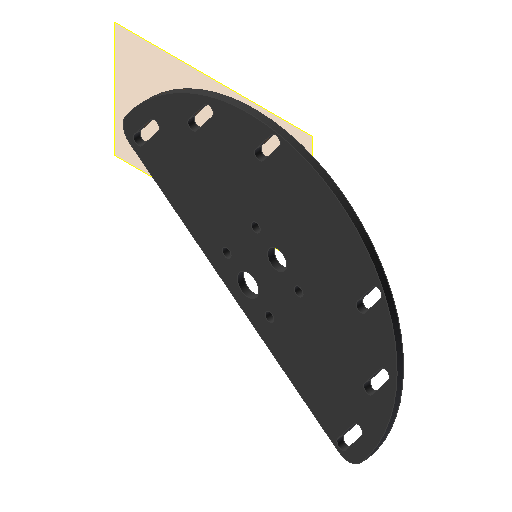
# Autodesk Inventor part: Anglerfish_Lightplate_Tosslink_adjuster_flipped
Saved by Autodesk Inventor 2022 (Build 260153000, 153)
## iProperties
Created: 2022-10-26
Part Number: Anglerfish_Lightplate_Tosslink_adjuster_flipped
Material: Generisch
Document SubType Name: Modeling
Designer: diederichbenedict
Density: 1 g/cm^3
Appearance: Vorgabe
Author: diederichbenedict
Autodesk Inventor part; units mm, degrees
ref_plane "YZ Plane" through (0, 0, 0) normal (1, 0, 0) x (0, 1, 0)
ref_plane "XZ Plane" through (0, 0, 0) normal (0, 1, 0) x (-1, 0, 0)
ref_plane "XY Plane" through (0, 0, 0) normal (0, 0, 1) x (1, 0, 0)
ref_plane "Arbeitsebene1" through (0, 0, 0) normal (0, 0, 1) x (1, 0, 0)
sketch "Skizze1" plane through (0, 0, 0) normal (0, 0, 1) x (1, 0, 0)
  line L0 (39.3233, 58.7442) -> (31.1975, 48.5587) projected
  arc A0 (20.3661, 6.7006) -> (31.1975, 48.5587) centre (0, 34.301) ccw projected
  line L1 (20.3661, 6.7006) -> (24.3422, 1.3125) projected
  arc A1 (24.3422, 1.3125) -> (31.7994, 0.6471) centre (28.3654, 4.2814) ccw projected
  arc A2 (31.7994, 0.6471) -> (39.3233, 58.7442) centre (0, 34.301) ccw projected
  circle A3 centre (37.5836, 49.0481) radius 1.4 projected
  circle A4 centre (39.9219, 28.2806) radius 1.4 projected
  circle A5 centre (31.5631, 9.1262) radius 1.4 projected
  line L2 (6.9617, 67.8882) -> (15.0883, 78.0746) projected
  arc A6 (15.0883, 78.0746) -> (-39.8826, 57.8205) centre (0, 34.301) ccw projected
  arc A7 (-39.8826, 57.8205) -> (-37.5755, 50.698) centre (-35.5757, 55.2807) ccw projected
  line L3 (-37.5755, 50.698) -> (-31.4381, 48.0198) projected
  arc A8 (6.9617, 67.8882) -> (-31.4381, 48.0198) centre (0, 34.301) ccw projected
  circle A9 centre (-31.5631, 59.4759) radius 1.4 projected
  circle A10 centre (-14.7471, 71.8847) radius 1.4 projected
  circle A11 centre (6.0205, 74.2229) radius 1.4 projected
  circle A12 centre (-0.002, 34.3021) radius 3.35 projected
  circle A13 centre (9.062, 45.6666) radius 3 projected
  circle A14 centre (2.4174, 50.9675) radius 1.9 projected
  circle A15 centre (15.7065, 40.3657) radius 1.9 projected
  circle A16 centre (6.6446, 29.0001) radius 1.9 projected
  circle A17 centre (-6.6446, 39.602) radius 1.9 projected
  line L4 (31.7994, 0.6471) -> (-40.3324, 56.8214)
  arc A18 (20.3661, 6.7006) -> (-31.4381, 48.0198) centre (0, 34.301) ccw projected
  arc A19 (31.7994, 0.6471) -> (-39.8826, 57.8205) centre (0, 34.301) ccw projected
  circle A20 centre (15.7065, 40.3657) radius 1.4
  circle A21 centre (6.6446, 29.0001) radius 1.4
  circle A22 centre (-6.6446, 39.602) radius 1.4
  circle A23 centre (2.4174, 50.9675) radius 1.4
  point P0 (0, 0)
  dimension "d2" = 2.8
  dimension "d3" = 2.8
  dimension "d4" = 2.8
  dimension "d5" = 2.8
  constraints: 4 centre point, 4 coincident, 2 end point, 1 point on circle
  measures "d2" diameter of A20
  measures "d3" diameter of A21
  measures "d4" diameter of A22
  measures "d5" diameter of A23
extrude "Extrusion1" add sketch "Skizze1" along normal blind 2 contours A2 L4 A0 L0 | L0 A18 L2 A19 | A0 L4 A8 A18 | L2 A8 L4 A7 A6 | A14 | A15 | A16 | A17
sketch "Skizze2" plane through (0, 0, 2) normal (0, 0, 1) x (1, 0, 0)
  arc A0 (31.7994, 0.6471) -> (-39.8826, 57.8205) centre (0, 34.301) ccw projected
  arc A1 (-39.8826, 57.8205) -> (-40.3324, 56.8214) centre (-35.5757, 55.2807) ccw projected
  line L0 (-40.3324, 56.8214) -> (31.7994, 0.6471) projected
  circle A2 centre (31.5631, 9.1262) radius 1.4 projected
  circle A3 centre (39.9219, 28.2806) radius 1.4 projected
  circle A4 centre (37.5836, 49.0481) radius 1.4 projected
  circle A5 centre (-31.5631, 59.4759) radius 1.4 projected
  circle A6 centre (-14.7471, 71.8847) radius 1.4 projected
  circle A7 centre (6.0205, 74.2229) radius 1.4 projected
  circle A8 centre (9.062, 45.6666) radius 3 projected
  circle A9 centre (-0.002, 34.3021) radius 3.35 projected
  circle A10 centre (15.7065, 40.3657) radius 1.4 projected
  circle A11 centre (2.4174, 50.9675) radius 1.4 projected
  circle A12 centre (-6.6446, 39.602) radius 1.4 projected
  circle A13 centre (6.6446, 29.0001) radius 1.4 projected
  line L1 (29.1054, 5.9703) -> (34.0209, 12.2821) construction
  circle A14 centre (31.5631, 9.1262) radius 1.4 projected
  line L2 (30.3283, 5.018) -> (35.2438, 11.3297)
  line L3 (32.798, 13.2345) -> (27.8825, 6.9227)
  arc A15 (27.8825, 6.9227) -> (30.3283, 5.018) centre (29.1054, 5.9703) ccw
  arc A16 (35.2438, 11.3297) -> (32.798, 13.2345) centre (34.0209, 12.2821) ccw
  line L4 (37.4642, 25.1247) -> (42.3796, 31.4365) construction
  line L5 (38.6871, 24.1723) -> (43.6025, 30.4841)
  line L6 (41.1567, 32.3888) -> (36.2413, 26.0771)
  arc A17 (36.2413, 26.0771) -> (38.6871, 24.1723) centre (37.4642, 25.1247) ccw
  arc A18 (43.6025, 30.4841) -> (41.1567, 32.3888) centre (42.3796, 31.4365) ccw
  line L7 (35.1259, 45.8922) -> (40.0413, 52.204) construction
  line L8 (36.3488, 44.9399) -> (41.2642, 51.2516)
  line L9 (38.8184, 53.1564) -> (33.903, 46.8446)
  arc A19 (33.903, 46.8446) -> (36.3488, 44.9399) centre (35.1259, 45.8922) ccw
  arc A20 (41.2642, 51.2516) -> (38.8184, 53.1564) centre (40.0413, 52.204) ccw
  line L10 (3.5627, 71.0671) -> (8.4782, 77.3788) construction
  line L11 (4.7857, 70.1147) -> (9.7011, 76.4265)
  line L12 (7.2553, 78.3312) -> (2.3398, 72.0194)
  arc A21 (2.3398, 72.0194) -> (4.7857, 70.1147) centre (3.5627, 71.0671) ccw
  arc A22 (9.7011, 76.4265) -> (7.2553, 78.3312) centre (8.4782, 77.3788) ccw
  line L13 (-17.2048, 68.7288) -> (-12.2894, 75.0405) construction
  line L14 (-15.9819, 67.7764) -> (-11.0664, 74.0882)
  line L15 (-13.5123, 75.9929) -> (-18.4277, 69.6811)
  arc A23 (-18.4277, 69.6811) -> (-15.9819, 67.7764) centre (-17.2048, 68.7288) ccw
  arc A24 (-11.0664, 74.0882) -> (-13.5123, 75.9929) centre (-12.2894, 75.0405) ccw
  line L16 (-34.0209, 56.32) -> (-29.1054, 62.6318) construction
  line L17 (-32.798, 55.3676) -> (-27.8825, 61.6794)
  line L18 (-30.3283, 63.5841) -> (-35.2438, 57.2723)
  arc A25 (-35.2438, 57.2723) -> (-32.798, 55.3676) centre (-34.0209, 56.32) ccw
  arc A26 (-27.8825, 61.6794) -> (-30.3283, 63.5841) centre (-29.1054, 62.6318) ccw
  line L19 (29.1054, 5.9703) -> (34.0209, 12.2821) construction
  line L20 (30.3283, 5.018) -> (35.2438, 11.3297)
  line L21 (32.798, 13.2345) -> (27.8825, 6.9227)
  arc A27 (27.8825, 6.9227) -> (30.3283, 5.018) centre (29.1054, 5.9703) ccw
  arc A28 (35.2438, 11.3297) -> (32.798, 13.2345) centre (34.0209, 12.2821) ccw
  point P0 (0, 0)
  dimension "d6" = 4
  dimension "d7" = 3.1
  dimension "d8" = 3.1
  dimension "d9" = 3.1
  dimension "d10" = 3.1
  dimension "d11" = 3.1
  dimension "d12" = 3.1
  dimension "d13" = 3.1
  constraints: 56 end point, 28 point on circle, 28 tangent, 14 centre point, 7 parallel, 1 midpoint
  measures "d6" distance of A14.centre L1.end
  measures "d7" diameter of A16
  measures "d8" diameter of A18
  measures "d9" diameter of A20
  measures "d10" diameter of A22
  measures "d11" diameter of A24
  measures "d12" diameter of A26
  measures "d13" diameter of A28
extrude "Extrusion2" cut sketch "Skizze2" against normal blind 2 contours A7 | A15 L3 A16 L2 | A17 L6 A18 L5 | A19 L9 A20 L8 | A21 L12 A22 L11 | A23 L15 A24 L14 | A25 L18 A26 L17
fillet "Rundung1" radius 5 2 edges at (-40.3324, 56.8214, 1) (31.7994, 0.6471, 1)
